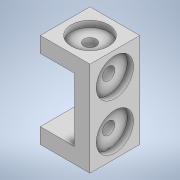
# Autodesk Inventor part: MountingBracket_Double
Saved by Autodesk Inventor 2020 (Build 240168000, 168)
## iProperties
Created: 2022-02-07
Part Number: MountingBracket_Double
Material: Generic
Document SubType Name: Modeling
Designer: danie
Density: 1 g/cm^3
Appearance: Default
Author: danie
Autodesk Inventor part; units mm, degrees
ref_plane "YZ Plane" through (0, 0, 0) normal (1, 0, 0) x (0, 1, 0)
ref_plane "XZ Plane" through (0, 0, 0) normal (0, 1, 0) x (-1, 0, 0)
ref_plane "XY Plane" through (0, 0, 0) normal (0, 0, 1) x (1, 0, 0)
sketch "Sketch1" plane through (0, 0, 0) normal (1, 0, 0) x (0, 1, 0)
  line L0 (0, 0) -> (48.26, 0)
  line L1 (48.26, 0) -> (48.26, -25.4)
  line L2 (48.26, -25.4) -> (0, -25.4)
  line L3 (0, -25.4) -> (0, 0)
  line L4 (0, 0) -> (24.13, 0) construction
  line L5 (24.13, 0) -> (24.13, -25.4) construction
  line L6 (24.13, -25.4) -> (0, -25.4) construction
  line L7 (0, -25.4) -> (0, 0) construction
  line L8 (24.13, 0) -> (0, -25.4) construction
  line L9 (0, 0) -> (24.13, -25.4) construction
  line L10 (24.13, 0) -> (48.26, -25.4) construction
  line L11 (48.26, 0) -> (24.13, -25.4) construction
  circle A0 centre (12.065, -12.7) radius 3.175
  circle A1 centre (36.195, -12.7) radius 3.175
  dimension "d0" = 48.26
  dimension "d1" = 25.4
  dimension "d2" = 24.13
  dimension "d3" = 25.4
  dimension "d32" = 6.35
  dimension "d33" = 6.35
  constraints: 24 end point, 4 parallel, 2 centre point, 2 horizontal, 2 midpoint, 2 perpendicular
  measures "d0" distance of L1.end L2.end
  measures "d1" distance of L0.end L1.end
  measures "d2" distance of L5.end L6.end
  measures "d3" distance of L4.end L5.end
  measures "d32" diameter of A0
  measures "d33" diameter of A1
extrude "Extrusion1" add sketch "Sketch1" against normal blind 7.9375
sketch "Sketch2" plane through (0, 48.26, 0) normal (0, 1, 0) x (1, 0, 0)
  line L0 (0, 0) -> (-25.4, 0)
  line L1 (-25.4, 0) -> (-25.4, 25.4)
  line L2 (-25.4, 25.4) -> (0, 25.4)
  line L3 (0, 25.4) -> (0, 0)
  line L4 (0, 0) -> (-7.9375, 0) construction
  line L5 (-25.4, 25.4) -> (0, 0) construction
  line L6 (0, 0) -> (0, 25.4) construction
  line L7 (0, 25.4) -> (-25.4, 0) construction
  circle A0 centre (-12.7, 12.7) radius 3.175
  dimension "d8" = 25.4
  dimension "d9" = 25.4
  dimension "d34" = 6.35
  constraints: 14 end point, 2 parallel, 2 perpendicular, 1 centre point, 1 horizontal, 1 midpoint
  measures "d8" distance of L1.end L2.end
  measures "d9" distance of L0.end L1.end
  measures "d34" diameter of A0
extrude "Extrusion2" add sketch "Sketch2" against normal blind 7.9375
sketch "Sketch5" plane through (-7.9375, 0, 0) normal (0, 0, 1) x (1, 0, 0)
  line L0 (7.9375, 0) -> (7.9375, 48.26) projected
  line L1 (7.9375, 0) -> (-17.4625, 0)
  line L2 (-17.4625, 0) -> (-17.4625, 7.9375)
  line L3 (-17.4625, 7.9375) -> (7.9375, 7.9375)
  line L4 (7.9375, 7.9375) -> (7.9375, 0)
  dimension "d19" = 25.4
  dimension "d20" = 7.9375
  constraints: 8 end point, 2 parallel, 1 horizontal, 1 perpendicular
  measures "d19" distance of L2.end L3.end
  measures "d20" distance of L1.end L2.end
extrude "Extrusion3" add sketch "Sketch5" against normal blind 25.4
sketch "Sketch6" plane through (0, 0, -25.4) normal (0, -1, 0) x (1, 0, 0)
  line L0 (-7.9375, 25.4) -> (-25.4, 25.4) construction
  line L1 (0, 0) -> (-25.4, 0) construction
  line L2 (-25.4, 25.4) -> (0, 0) construction
  line L3 (0, 0) -> (0, 25.4) construction
  line L4 (-25.4, 0) -> (0, 25.4) construction
  circle A0 centre (-12.7, 12.7) radius 3.175
  dimension "d35" = 6.35
  constraints: 4 end point, 1 centre point, 1 midpoint
  measures "d35" diameter of A0
sketch "Sketch7" plane through (0, 0, 0) normal (1, 0, 0) x (0, 0, -1)
  line L0 (0, 0) -> (25.4, 0) construction
  line L1 (25.4, 0) -> (25.4, 24.13) construction
  line L2 (25.4, 24.13) -> (0, 24.13) construction
  line L3 (0, 24.13) -> (0, 0) construction
  line L4 (0, 0) -> (25.4, 24.13) construction
  line L5 (0, 24.13) -> (25.4, 0) construction
  line L6 (0, 24.13) -> (25.4, 48.26) construction
  line L7 (25.4, 48.26) -> (0, 48.26) construction
  line L8 (25.4, 24.13) -> (0, 48.26) construction
  circle A0 centre (12.7, 12.065) radius 9.525
  circle A1 centre (12.7, 36.195) radius 9.525
  dimension "d26" = 25.4
  dimension "d27" = 24.13
  dimension "d28" = 19.05
  dimension "d29" = 19.05
  constraints: 16 end point, 2 centre point, 2 midpoint, 2 parallel, 1 horizontal, 1 perpendicular
  measures "d26" distance of L2.end L1.end
  measures "d27" distance of L1.end L0.end
  measures "d28" diameter of A0
  measures "d29" diameter of A1
extrude "Extrusion5" cut sketch "Sketch7" against normal blind 3.175
extrude "Extrusion6" cut sketch "Sketch6" against normal blind 7.9375
sketch "Sketch8" plane through (0, 0, -25.4) normal (0, -1, 0) x (1, 0, 0)
  line L0 (-7.9375, 25.4) -> (-25.4, 25.4) construction
  line L1 (0, 0) -> (-25.4, 0) construction
  line L2 (-25.4, 25.4) -> (0, 0) construction
  line L3 (0, 0) -> (0, 25.4) construction
  line L4 (-25.4, 25.4) -> (-25.4, 0) construction
  line L5 (0, 25.4) -> (-25.4, 0) construction
  circle A0 centre (-12.7, 12.7) radius 9.525
  dimension "d38" = 19.05
  constraints: 6 end point, 2 perpendicular, 1 centre point, 1 midpoint
  measures "d38" diameter of A0
extrude "Extrusion7" cut sketch "Sketch8" against normal blind 3.175
sketch "Sketch9" plane through (0, 48.26, 0) normal (0, 1, 0) x (1, 0, 0)
  line L0 (-25.4, 25.4) -> (-7.9375, 25.4) construction
  line L1 (0, 0) -> (-25.4, 25.4) construction
  line L2 (-7.9375, 0) -> (-25.4, 0) construction
  line L3 (0, 25.4) -> (-25.4, 25.4) construction
  line L4 (-25.4, 0) -> (0, 25.4) construction
  circle A0 centre (-12.7, 12.7) radius 9.525
  dimension "d41" = 19.05
  constraints: 4 end point, 1 centre point, 1 midpoint
  measures "d41" diameter of A0
extrude "Extrusion8" cut sketch "Sketch9" against normal blind 3.175
body "Solid1"
